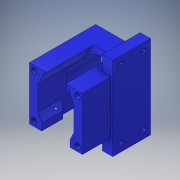
# Autodesk Inventor part: Upper_Unit
Saved by Autodesk Inventor 2019 (Build 230136000, 136)
## iProperties
Created: 2018-10-10
Part Number: Upper_Unit
Material: Generisch
Document SubType Name: Modeling
Designer: janbe
Density: 1 g/cm^3
Appearance: Blau - Wandfarbe - glänzend
Author: janbe
Autodesk Inventor part; units mm, degrees
ref_plane "YZ Plane" through (0, 0, 0) normal (1, 0, 0) x (0, 1, 0)
ref_plane "XZ Plane" through (0, 0, 0) normal (0, 1, 0) x (-1, 0, 0)
ref_plane "XY Plane" through (0, 0, 0) normal (0, 0, 1) x (1, 0, 0)
sketch "Skizze1" plane through (0, 0, 0) normal (0, 0, 1) x (1, 0, 0)
  line L0 (-14, -14) -> (14, -14)
  line L1 (14, -14) -> (14, 14)
  line L2 (14, 14) -> (-14, 14)
  line L3 (-14, 14) -> (-14, -14)
  line L4 (-14, -14) -> (14, 14) construction
  line L5 (14, -14) -> (-14, 14) construction
  circle A0 centre (-11.5, 11.5) radius 1.5
  circle A1 centre (11.5, 11.5) radius 1.5
  circle A2 centre (-11.5, -11.5) radius 1.5
  circle A3 centre (11.5, -11.5) radius 1.5
  point P0 (0, 0)
  dimension "d0" = 28
  dimension "d1" = 28
  dimension "d4" = 3
  dimension "d5" = 2.5
  dimension "d6" = 2.5
  dimension "d9" = 23
  dimension "d12" = 23
  constraints: 12 end point, 4 centre point, 2 horizontal, 2 midpoint, 2 parallel, 1 perpendicular, 1 point on line, 1 vertical, 6 other
  measures "d0" distance of L2.end L1.end
  measures "d1" distance of L1.end L0.end
  measures "d4" diameter of A0
  measures "d5" distance from line of L2 A0.centre
  measures "d6" distance from line of A0.centre L3
  measures "d9" distance of A0.centre A1.centre
  measures "d12" distance of A0.centre A2.centre
extrude "Extrusion2" add sketch "Skizze1" along normal blind 5
sketch "Skizze2" plane through (0, 0, 0) normal (0, 0, -1) x (-1, 0, 0)
  circle A0 centre (0, 0) radius 6 projected
  line L0 (9.35, 6.25) -> (6.6987, 11.6324) projected
  arc A1 (6.6987, 11.6324) -> (-6.6987, 11.6324) centre (0, 8.3327) ccw projected
  line L1 (-6.6987, 11.6324) -> (-9.35, 6.25) projected
  line L2 (-9.35, 6.25) -> (-9.35, -6.25) projected
  line L3 (-9.35, -6.25) -> (-6.6987, -11.6324) projected
  arc A2 (-6.6987, -11.6324) -> (6.6987, -11.6324) centre (0, -8.3327) ccw projected
  line L4 (6.6987, -11.6324) -> (9.35, -6.25) projected
  line L5 (9.35, -6.25) -> (9.35, 6.25) projected
  circle A3 centre (-11.5, -11.5) radius 1.5 projected
  circle A4 centre (11.5, -11.5) radius 1.5 projected
  circle A5 centre (-11.5, 11.5) radius 1.5 projected
  circle A6 centre (11.5, 11.5) radius 1.5 projected
  line L6 (14, -14) -> (-14, -14) projected
  line L7 (14, 14) -> (14, -14) projected
  line L8 (-14, 14) -> (14, 14) projected
  line L9 (-14, -14) -> (-14, 14) projected
  line L10 (-9.5, -6.3503) -> (-9.5, 6.3503)
  line L11 (-9.5, 6.3503) -> (-6.8061, 11.819)
  line L12 (6.8061, 11.819) -> (9.5, 6.3503)
  line L13 (9.5, -6.3503) -> (9.5, 6.3503)
  line L14 (9.5, -6.3503) -> (6.8061, -11.819)
  line L15 (-9.5, -6.3503) -> (-6.8061, -11.819)
  arc A7 (-6.8061, -11.819) -> (6.8061, -11.819) centre (0, -8.4664) ccw
  arc A8 (6.8061, 11.819) -> (-6.8061, 11.819) centre (0, 8.4664) ccw
  point P0 (0, 0)
  dimension "d77" = 19
  constraints: 12 end point, 6 parallel, 4 point on circle, 2 centre point
  measures "d77" distance between parallel lines of L10 L13
extrude "Extrusion3" cut sketch "Skizze2" against normal up to surface (5 mm away) contours A0 | L5 L4 A2 L6 L3 L2 L1 A1 L8 L0 | L0 A1 L8 A8 L12 L13 L14 A7 L6 A2 L4 L5 | L8 A1 | A1 L8 A8 | A1 L1 L2 L3 A2 L6 A7 L15 L10 L11 A8 L8 | L6 A7 A2 | A2 L6
sketch "Skizze4" plane through (0, 0, 0) normal (0, 0, -1) x (-1, 0, 0)
  arc A0 (-6.8061, -11.819) -> (-5.1907, -14) centre (0, -8.4664) ccw projected
  line L0 (-6.8061, -11.819) -> (-9.5, -6.3503) projected
  line L1 (-9.5, -6.3503) -> (-9.5, 6.3503) projected
  line L2 (-9.5, 6.3503) -> (-6.8061, 11.819) projected
  arc A1 (-5.1907, 14) -> (-6.8061, 11.819) centre (0, 8.4664) ccw projected
  line L3 (-14, 14) -> (-5.1907, 14) projected
  line L4 (-14, -14) -> (-14, 14) projected
  line L5 (-5.1907, -14) -> (-14, -14) projected
  circle A2 centre (-11.5, 11.5) radius 1.5 projected
  circle A3 centre (-11.5, -11.5) radius 1.5 projected
  arc A4 (5.1907, -14) -> (6.8061, -11.819) centre (0, -8.4664) ccw projected
  line L6 (14, -14) -> (5.1907, -14) projected
  line L7 (14, 14) -> (14, -14) projected
  line L8 (5.1907, 14) -> (14, 14) projected
  arc A5 (6.8061, 11.819) -> (5.1907, 14) centre (0, 8.4664) ccw projected
  line L9 (6.8061, 11.819) -> (9.5, 6.3503) projected
  line L10 (9.5, 6.3503) -> (9.5, -6.3503) projected
  line L11 (9.5, -6.3503) -> (6.8061, -11.819) projected
  circle A6 centre (11.5, -11.5) radius 1.5 projected
  circle A7 centre (11.5, 11.5) radius 1.5 projected
  line L12 (14, -14) -> (5.1907, -14) projected
  line L13 (14, 14) -> (9.5, 14)
  line L14 (9.5, 14) -> (9.5, -14)
  line L15 (9.5, -14) -> (14, -14)
  line L16 (14, -14) -> (14, 14)
  line L17 (-14, 14) -> (-5.1907, 14) projected
  line L18 (-14, -14) -> (-9.5, -14)
  line L19 (-9.5, -14) -> (-9.5, 14)
  line L20 (-9.5, 14) -> (-14, 14)
  line L21 (-14, 14) -> (-14, -14)
  line L22 (-9.5, -6.3503) -> (-9.5, 6.3503) projected
  line L23 (9.5, 6.3503) -> (9.5, -6.3503) projected
  point P0 (0, 0)
  constraints: 16 end point, 4 parallel, 2 collinear, 2 horizontal, 2 perpendicular, 2 point on line
extrude "Extrusion4" add sketch "Skizze4" along normal blind 30
sketch "Skizze5" plane through (0, 0, -30) normal (0, 0, -1) x (-1, 0, 0)
  circle A0 centre (-11.5, -11.5) radius 1.5 projected
  circle A1 centre (-11.5, 11.5) radius 1.5 projected
  line L0 (-5.1907, 14) -> (-14, 14) projected
  line L1 (-14, 14) -> (-14, -14) projected
  line L2 (-14, -14) -> (-5.1907, -14) projected
  arc A2 (-6.8061, -11.819) -> (-5.1907, -14) centre (0, -8.4664) ccw projected
  line L3 (-6.8061, -11.819) -> (-9.5, -6.3503) projected
  line L4 (-9.5, -6.3503) -> (-9.5, 6.3503) projected
  line L5 (-9.5, 6.3503) -> (-6.8061, 11.819) projected
  arc A3 (-5.1907, 14) -> (-6.8061, 11.819) centre (0, 8.4664) ccw projected
  circle A4 centre (11.5, 11.5) radius 1.5 projected
  circle A5 centre (11.5, -11.5) radius 1.5 projected
  arc A6 (5.1907, -14) -> (6.8061, -11.819) centre (0, -8.4664) ccw projected
  line L6 (5.1907, -14) -> (14, -14) projected
  line L7 (14, -14) -> (14, 14) projected
  line L8 (14, 14) -> (5.1907, 14) projected
  arc A7 (6.8061, 11.819) -> (5.1907, 14) centre (0, 8.4664) ccw projected
  line L9 (6.8061, 11.819) -> (9.5, 6.3503) projected
  line L10 (9.5, 6.3503) -> (9.5, -6.3503) projected
  line L11 (9.5, -6.3503) -> (6.8061, -11.819) projected
  line L12 (-9.5, -6.3503) -> (-9.5, -14)
  line L13 (9.5, -6.3503) -> (9.5, 6.3503) projected
  line L14 (9.5, -6.3503) -> (9.5, -14)
  line L15 (-9.5, -6.3503) -> (-9.5, 6.3503) projected
  point P0 (0, 0)
  constraints: 4 end point, 2 collinear, 2 point on line
extrude "Extrusion5" cut sketch "Skizze5" against normal blind 25 contours L12 L3 A2 L2 | A6 L11 L14 L6
sketch "Skizze6" plane through (0, 0, -30) normal (0, 0, -1) x (-1, 0, 0)
  line L0 (-9.5, -14) -> (-9.5, 6.3503) projected
  line L1 (-9.5, 6.3503) -> (-6.8061, 11.819) projected
  arc A0 (-5.1907, 14) -> (-6.8061, 11.819) centre (0, 8.4664) ccw projected
  line L2 (-5.1907, 14) -> (-14, 14) projected
  line L3 (-14, 14) -> (-14, -14) projected
  line L4 (-14, -14) -> (-9.5, -14) projected
  circle A1 centre (-11.5, 11.5) radius 1.5 projected
  circle A2 centre (-11.5, -11.5) radius 1.5 projected
  line L5 (9.5, 6.3503) -> (9.5, -14) projected
  line L6 (9.5, -14) -> (14, -14) projected
  line L7 (14, -14) -> (14, 14) projected
  line L8 (14, 14) -> (5.1907, 14) projected
  arc A3 (6.8061, 11.819) -> (5.1907, 14) centre (0, 8.4664) ccw projected
  line L9 (6.8061, 11.819) -> (9.5, 6.3503) projected
  circle A4 centre (11.5, -11.5) radius 1.5 projected
  circle A5 centre (11.5, 11.5) radius 1.5 projected
  line L10 (-9.5, -14) -> (9.5, -14)
  line L11 (14, -14) -> (5.1907, -14) projected
  line L12 (-5.1907, 14) -> (5.1907, 14)
  circle A6 centre (0, 0) radius 11
  dimension "d25" = 22
  constraints: 4 end point, 1 centre point, 1 coincident, 1 collinear, 1 parallel
  measures "d25" diameter of A6
extrude "Extrusion6" add sketch "Skizze6" against normal blind 20 contours L0 A6 L5 L10 | L0 A6 L5 | L0 L1 A0 L12 A3 L9 L5 A6
sketch "Skizze7" plane through (0, 0, -30) normal (0, 0, -1) x (-1, 0, 0)
  circle A0 centre (0, 0) radius 11.1
  dimension "d26" = 22.2
  constraints: 1 centre point, 1 coincident
  measures "d26" diameter of A0
extrude "Extrusion7" cut sketch "Skizze7" against normal up to surface (20 mm away)
sketch "Skizze9" plane through (14, -14, 5) normal (1, 0, 0) x (0, 0, -1)
  line L0 (35, 28) -> (0, 28) projected
  line L1 (0, 0) -> (0, 28) projected
  line L2 (35, 0) -> (0, 0) projected
  line L3 (35, 28) -> (35, 0) projected
  line L4 (35, -8) -> (15, -8)
  line L5 (15, -8) -> (15, 36)
  line L6 (15, 36) -> (35, 36)
  line L7 (35, 36) -> (35, -8)
  circle A0 centre (31, 32) radius 1.5
  circle A1 centre (31, -4) radius 1.5
  circle A2 centre (19, 32) radius 1.5
  circle A3 centre (19, -4) radius 1.5
  line L8 (0, 0) -> (15, 0) projected
  line L9 (35, 28) -> (15, 28)
  line L10 (15, 28) -> (15, 0)
  line L11 (15, 0) -> (35, 0)
  line L12 (35, 0) -> (35, 28)
  point P0 (10, 0)
  dimension "d29" = 20
  dimension "d30" = 8
  dimension "d31" = 8
  dimension "d32" = 3
  dimension "d33" = 4
  dimension "d34" = 4
  dimension "d37" = 36
  dimension "d40" = 12
  constraints: 16 end point, 4 centre point, 4 parallel, 3 horizontal, 2 perpendicular, 1 collinear, 1 vertical, 6 other
  measures "d29" distance of L5.end L6.end
  measures "d30" distance between parallel lines of L0 L6
  measures "d31" distance between parallel lines of L4 L2
  measures "d32" diameter of A0
  measures "d33" distance from line of L6 A0.centre
  measures "d34" distance from line of L7 A0.centre
  measures "d37" distance of A0.centre A1.centre
  measures "d40" distance of A0.centre A2.centre
extrude "Extrusion8" add sketch "Skizze9" against normal up to surface (4.5 mm away) contours L0 L5 L6 L7 | L7 L4 L5 L2
chamfer "Fase1" distance 3.9 angle 30 1 edges at (-9.5, -10.1751, -5) measured on face at (-9, -10.1751, -5)
chamfer "Fase2" distance 3.9 angle 30 1 edges at (9.5, -10.1751, -5) measured on face at (9, -10.1751, -5)
sketch "Skizze11" plane through (14, -14, 5) normal (1, 0, 0) x (0, 0, -1)
  circle A0 centre (31, -4) radius 1.5 projected
  circle A1 centre (19, -4) radius 1.5 projected
  circle A2 centre (19, 32) radius 1.5 projected
  circle A3 centre (31, 32) radius 1.5 projected
  line L0 (15, 28) -> (0, 28) projected
  line L1 (0, 0) -> (0, 28) projected
  line L2 (15, 0) -> (0, 0) projected
  line L3 (15, 28) -> (15, 36) projected
  line L4 (35, -8) -> (15, -8) projected
  line L5 (35, 36) -> (35, -8) projected
  line L6 (15, 36) -> (35, 36) projected
  line L7 (35, 36) -> (35, -8) projected
  line L8 (15, -8) -> (15, 36) projected
  line L9 (35, 36) -> (15, 36)
  line L10 (15, 36) -> (15, -8)
  line L11 (15, -8) -> (35, -8)
  line L12 (35, -8) -> (35, 36)
  line L13 (15, -8) -> (15, 0) projected
  point P0 (5, 14)
  constraints: 8 end point, 2 parallel, 1 horizontal, 1 perpendicular
extrude "Extrusion10" add sketch "Skizze11" along normal blind 1 contours L3 L6 L5 L4 L8
sketch "Skizze12" plane through (0, 0, -10) normal (0, 0, 1) x (1, 0, 0)
  point P0 (0, 0)
sketch "Skizze13" plane through (9.5, -22, -30) normal (-1, 0, 0) x (0, 0, 1)
  circle A0 centre (4, 4) radius 1.5 projected
  circle A1 centre (16, 4) radius 1.5 projected
  line L0 (0, 8) -> (20, 8) projected
  line L1 (0, 8) -> (0, 0) projected
  line L2 (0, 0) -> (20, 0) projected
  line L3 (20, 0) -> (20, 8) projected
  circle A2 centre (16, 40) radius 1.5 projected
  circle A3 centre (4, 40) radius 1.5 projected
  line L4 (20, 36) -> (20, 44) projected
  line L5 (20, 44) -> (0, 44) projected
  line L6 (0, 44) -> (0, 36) projected
  line L7 (20, 36) -> (0, 36) projected
  line L8 (4, 0.94) -> (1.35, 2.47)
  line L9 (1.35, 2.47) -> (1.35, 5.53)
  line L10 (1.35, 5.53) -> (4, 7.06)
  line L11 (4, 7.06) -> (6.65, 5.53)
  line L12 (6.65, 5.53) -> (6.65, 2.47)
  line L13 (6.65, 2.47) -> (4, 0.94)
  line L14 (13.35, 5.53) -> (16, 7.06)
  line L15 (16, 7.06) -> (18.65, 5.53)
  line L16 (13.35, 2.47) -> (13.35, 5.53)
  line L17 (18.65, 5.53) -> (18.65, 2.47)
  line L18 (18.65, 2.47) -> (16, 0.94)
  line L19 (16, 0.94) -> (13.35, 2.47)
  line L20 (1.35, 41.53) -> (4, 43.06)
  line L21 (4, 43.06) -> (6.65, 41.53)
  line L22 (1.35, 38.47) -> (1.35, 41.53)
  line L23 (6.65, 41.53) -> (6.65, 38.47)
  line L24 (6.65, 38.47) -> (4, 36.94)
  line L25 (4, 36.94) -> (1.35, 38.47)
  line L26 (13.35, 41.53) -> (16, 43.06)
  line L27 (16, 43.06) -> (18.65, 41.53)
  line L28 (13.35, 38.47) -> (13.35, 41.53)
  line L29 (18.65, 41.53) -> (18.65, 38.47)
  line L30 (18.65, 38.47) -> (16, 36.94)
  line L31 (16, 36.94) -> (13.35, 38.47)
  point P0 (30, 22)
  point P1 (16, 4)
  point P2 (4, 40)
  point P3 (16, 40)
  dimension "d64" = 5.3
  dimension "d67" = 12
  dimension "d70" = 36
  constraints: 48 end point, 1 coincident, 1 horizontal, 1 parallel, 1 vertical, 52 other
  measures "d64" distance between parallel lines of L9 L12
  measures "d67" distance of L10.end L14.end
  measures "d70" distance of L10.end L20.end
extrude "Extrusion11" cut sketch "Skizze13" against normal blind 2 contours L8 L9 L10 L11 L12 L13 | L14 L15 L17 L18 L19 L16 | L20 L21 L23 L24 L25 L22 | L26 L27 L29 L30 L31 L28
sketch "Skizze14" plane through (0, 0, -10) normal (0, 0, 1) x (1, 0, 0)
  arc A0 (-9.5, -5.7411) -> (9.5, -5.7411) centre (0, 0) ccw projected
  line L0 (-9.5, -14) -> (-9.5, -5.7411) projected
  line L1 (-9.5, -14) -> (9.5, -14) projected
  line L2 (9.5, -5.7411) -> (9.5, -14) projected
  arc A1 (9.5, 5.7411) -> (-9.5, 5.7411) centre (0, 0) ccw projected
  line L3 (9.5, 6.3503) -> (9.5, 5.7411) projected
  line L4 (6.8061, 11.819) -> (9.5, 6.3503) projected
  arc A2 (6.8061, 11.819) -> (5.1907, 14) centre (0, 8.4664) ccw projected
  line L5 (5.1907, 14) -> (-5.1907, 14) projected
  arc A3 (-5.1907, 14) -> (-6.8061, 11.819) centre (0, 8.4664) ccw projected
  line L6 (-9.5, 6.3503) -> (-6.8061, 11.819) projected
  line L7 (-9.5, 5.7411) -> (-9.5, 6.3503) projected
extrude "Extrusion12" cut sketch "Skizze14" against normal blind 10
sketch "Skizze15" plane through (0, 0, 5) normal (0, 0, 1) x (1, 0, 0)
  point P0 (0, 0)
sketch "Skizze16" plane through (0, 0, 5) normal (0, 0, 1) x (1, 0, 0)
  arc A0 (5.1907, -14) -> (6.8061, -11.819) centre (0, -8.4664) ccw projected
  line L0 (5.1907, -14) -> (14, -14) projected
  line L1 (14, -14) -> (14, 14) projected
  line L2 (14, 14) -> (5.1907, 14) projected
  arc A1 (6.8061, 11.819) -> (5.1907, 14) centre (0, 8.4664) ccw projected
  line L3 (6.8061, 11.819) -> (9.5, 6.3503) projected
  line L4 (9.5, 6.3503) -> (9.5, -6.3503) projected
  line L5 (9.5, -6.3503) -> (6.8061, -11.819) projected
  circle A2 centre (11.5, -11.5) radius 1.5 projected
  circle A3 centre (11.5, 11.5) radius 1.5 projected
  arc A4 (-6.8061, -11.819) -> (-5.1907, -14) centre (0, -8.4664) ccw projected
  line L6 (-6.8061, -11.819) -> (-9.5, -6.3503) projected
  line L7 (-9.5, -6.3503) -> (-9.5, 6.3503) projected
  line L8 (-9.5, 6.3503) -> (-6.8061, 11.819) projected
  arc A5 (-5.1907, 14) -> (-6.8061, 11.819) centre (0, 8.4664) ccw projected
  line L9 (-5.1907, 14) -> (-14, 14) projected
  line L10 (-14, 14) -> (-14, -14) projected
  line L11 (-14, -14) -> (-5.1907, -14) projected
  circle A6 centre (-11.5, 11.5) radius 1.5 projected
  circle A7 centre (-11.5, -11.5) radius 1.5 projected
  line L12 (7.5, -14) -> (-7.5, -14)
  line L13 (-7.5, -14) -> (-7.5, -4)
  line L14 (-7.5, -4) -> (7.5, -4)
  line L15 (7.5, -4) -> (7.5, -14)
  point P0 (0, 0)
  dimension "d78" = 15
  dimension "d79" = 7.5
  dimension "d80" = 10
  constraints: 8 end point, 2 parallel, 1 horizontal, 1 perpendicular, 1 point on line
  measures "d78" distance of L13.end L14.end
  measures "d79" distance from line of point (0, 0) L15
  measures "d80" distance of L12.end L13.end
extrude "Extrusion13" cut sketch "Skizze16" against normal up to surface (25 mm away) contours L12 A4 L6 L13 L14 L15 L5 A0 | A0 L5 L15 L0 | L11 L13 L6 A4
